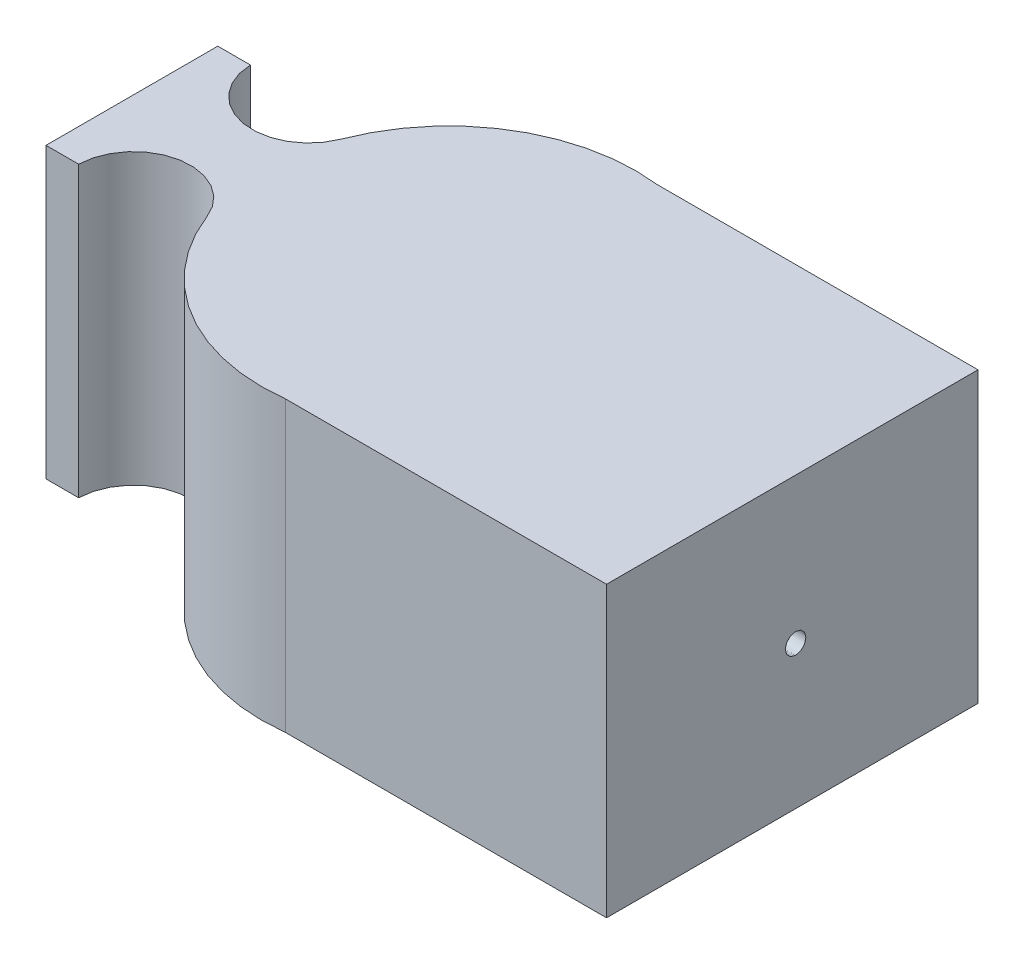
# Autodesk Inventor part: Durometer_Sensor
Saved by Autodesk Inventor 2015 SP1 (Build 190203100, 203)
## iProperties
Created: 2014-12-16
Part Number: Durometer_Sensor
Material: Generic
Document SubType Name: Modeling
Designer: Drew
Density: 1 g/cm^3
Appearance: Anodized - Blue
Author: Drew
Autodesk Inventor part; units mm, degrees
ref_plane "YZ Plane" through (0, 0, 0) normal (1, 0, 0) x (0, 1, 0)
ref_plane "XZ Plane" through (0, 0, 0) normal (0, 1, 0) x (-1, 0, 0)
ref_plane "XY Plane" through (0, 0, 0) normal (0, 0, 1) x (1, 0, 0)
sketch "Sketch1" plane through (0, 0, 0) normal (0, 1, 0) x (-1, 0, 0)
  line L0 (-24.6998, -28.575) -> (24.6998, -28.575)
  line L1 (24.6998, 28.575) -> (-24.6998, 28.575)
  line L2 (-24.6998, 28.575) -> (-24.6998, -28.575)
  line L3 (-24.6998, -28.575) -> (24.6998, 28.575) construction
  line L4 (24.6998, -28.575) -> (-24.6998, 28.575) construction
  arc A0 (55.0184, 10.3359) -> (71.8794, 13.215) centre (63.1598, 13.4684) ccw
  line L5 (74.3603, 0) -> (-43.8805, 0)
  arc A1 (71.8794, -13.215) -> (55.0184, -10.3359) centre (63.1598, -13.4684) ccw
  line L6 (71.8794, 13.215) -> (76.9002, 13.215)
  line L7 (76.9002, 13.215) -> (76.9002, -13.215)
  line L8 (76.9002, -13.215) -> (71.8794, -13.215)
  arc A2 (55.0184, 10.3359) -> (24.6998, 28.575) centre (28.155, 0) ccw
  arc A3 (24.6998, -28.575) -> (55.0184, -10.3359) centre (28.155, 0) ccw
  point P0 (0, 0)
  dimension "d1" = 57.15
  dimension "d2" = 101.6
  constraints: 18 end point, 8 point on circle, 4 centre point, 3 horizontal, 2 midpoint, 2 parallel, 2 tangent, 1 perpendicular, 1 point on line, 1 symmetric about line, 4 other
  measures "d1" distance of L1.end L0.start
  measures "d2" distance between parallel lines of L7 L2
extrude "Extrusion1" add sketch "Sketch1" along normal blind 44.45
hole "Hole1" at (24.6998, 22.0232, -0.5107) direction (-1, 0, 0) diameter 3.175 depth 25.4 tip angle 118
body "Solid1"
